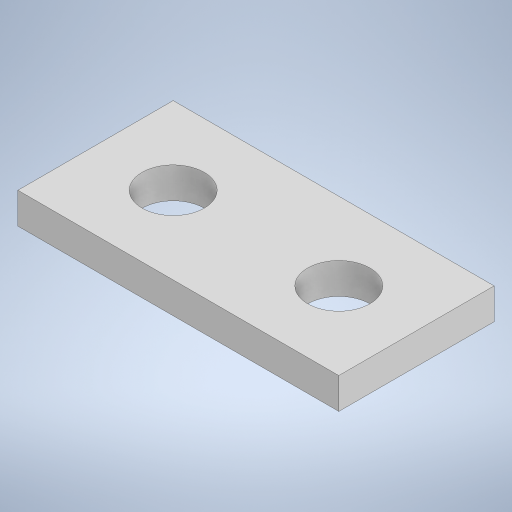
# Autodesk Inventor part: connector
Saved by Autodesk Inventor 2024 (Build 280153000, 153)
## iProperties
Created: 2023-11-20
Part Number: connector
Material: Generic
Document SubType Name: Modeling
Designer: olson
Density: 1 g/cm^3
Appearance: Default
Author: olson
Autodesk Inventor part; units mm, degrees
ref_plane "YZ Plane" through (0, 0, 0) normal (1, 0, 0) x (0, 1, 0)
ref_plane "XZ Plane" through (0, 0, 0) normal (0, 1, 0) x (-1, 0, 0)
ref_plane "XY Plane" through (0, 0, 0) normal (0, 0, 1) x (1, 0, 0)
sketch "Sketch1" plane through (0, 0, 0) normal (0, 1, 0) x (-1, 0, 0)
  line L0 (0, 0) -> (16, 0)
  line L1 (16, 0) -> (16, -8)
  line L2 (16, -8) -> (0, -8)
  line L3 (0, -8) -> (0, 0)
  dimension "d0" = 16
  dimension "d1" = 8
  constraints: 8 end point, 2 parallel, 1 horizontal, 1 perpendicular
  measures "d0" distance of L1.end L2.end
  measures "d1" distance of L0.end L1.end
extrude "Extrusion1" add sketch "Sketch1" along normal blind 1.5
sketch "Sketch2" plane through (0, 1.5, 0) normal (0, 1, 0) x (1, 0, 0)
  circle A0 centre (-4, 4) radius 1.5
  circle A1 centre (-12, 4) radius 1.5
  point P0 (0, 0)
  point P1 (-16, 0)
  dimension "d4" = 3
  dimension "d5" = 3
  constraints: 2 centre point
  measures "d4" diameter of A0
  measures "d5" diameter of A1
extrude "Extrusion2" cut sketch "Sketch2" against normal blind 1.5
sketch "Sketch3" plane through (0, 1.5, 0) normal (0, 1, 0) x (1, 0, 0)
  line L0 (-16, 0) -> (0, 0) projected
  line L1 (0, 0) -> (0, 8) projected
  line L2 (-16, 0) -> (0, 0)
  line L3 (0, 0) -> (0, 8)
  line L4 (0, 8) -> (-16, 8)
  line L5 (-16, 8) -> (-16, 0)
  line L6 (0, 0) -> (-0.25, 0)
  line L7 (-0.25, 0) -> (-0.25, 8)
  line L8 (0, 0) -> (0, 0.25)
  line L9 (0, 0.25) -> (-16, 0.25)
  line L10 (-16, 0) -> (-15.75, 0)
  line L11 (-15.75, 0) -> (-15.75, 8)
  line L12 (-16, 8) -> (-16, 7.75)
  line L13 (-16, 7.75) -> (-0.25, 7.75)
  point P0 (-0.25, 0.25)
  point P1 (-15.75, 0.25)
  point P2 (-15.75, 7.75)
  dimension "d8" = 0.25
  dimension "d9" = 0.25
  dimension "d10" = 0.25
  dimension "d11" = 0.25
  constraints: 24 end point, 8 point on line, 4 perpendicular, 3 parallel, 1 horizontal
  measures "d8" distance of L2.end L6.end
  measures "d9" distance of L2.end L8.end
  measures "d10" distance of L0.start L10.end
  measures "d11" distance of L4.end L12.end
extrude "Extrusion3" cut sketch "Sketch3" against normal blind 1.5 contours L5 L9 L11 L0 | L11 L9 L7 L0 | L5 L13 L11 L9 | L7 L9 L1 L0 | L5 L4 L11 L13 | L7 L4 L1 L9 | L11 L4 L7 L13
body "Solid1"
